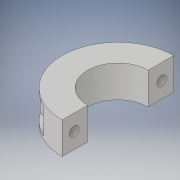
# Autodesk Inventor part: 000.402 - Зажим подшипника
Saved by Autodesk Inventor 2019 (Build 230136000, 136)
## iProperties
Created: 2020-02-28
Part Number: 000.402 - Зажим подшипника
Material: Типовые
Document SubType Name: Modeling
Designer: Петров Иван
Density: 1 g/cm^3
Appearance: По умолчанию
Author: Петров Иван
Autodesk Inventor part; units mm, degrees
ref_plane "YZ Plane" through (0, 0, 0) normal (1, 0, 0) x (0, 1, 0)
ref_plane "XZ Plane" through (0, 0, 0) normal (0, 1, 0) x (-1, 0, 0)
ref_plane "XY Plane" through (0, 0, 0) normal (0, 0, 1) x (1, 0, 0)
sketch "Эскиз1" plane through (0, 0, 0) normal (0, 1, 0) x (-1, 0, 0)
  circle A0 centre (0, 0) radius 9.5
  line L0 (0, -9.5) -> (0, -17.5)
  arc A1 (-7.7, -15.715) -> (-7.7, 15.715) centre (0, 0) ccw
  line L1 (0, 9.5) -> (0, 17.5)
  point P0 (0, -10)
  constraints: 6 point on circle, 4 end point, 2 centre point, 1 point on line
extrude "Выдавливание1" add sketch "Эскиз1" along normal blind 10 contours A0 L1 A1 L0
sketch "Эскиз2" plane through (0, 0, 17.5) normal (1, 0, 0) x (0, 0, -1)
  circle A0 centre (3.75, 5) radius 1.5 projected
  circle A1 centre (31.25, 5) radius 1.5 projected
  point P0 (17.5, 0)
extrude "Выдавливание2" cut sketch "Эскиз2" against normal through all
ref_plane "РабПлоскость1" through (-17.5, 0, 0) normal (1, 0, 0) x (0, 1, 0)
sketch "Эскиз3" plane through (-17.5, 0, 0) normal (1, 0, 0) x (0, 1, 0)
  line L0 (1, -17.25) -> (9, -17.25)
  line L1 (9, -17.25) -> (9, -10.25)
  line L2 (9, -10.25) -> (1, -10.25)
  line L3 (1, -10.25) -> (1, -17.25)
  circle A0 centre (5, -13.75) radius 1.5 projected
  line L4 (1, -17.25) -> (9, -10.25) construction
  line L5 (9, -17.25) -> (1, -10.25) construction
  line L6 (1, 10.25) -> (9, 10.25)
  line L7 (9, 10.25) -> (9, 17.25)
  line L8 (9, 17.25) -> (1, 17.25)
  line L9 (1, 17.25) -> (1, 10.25)
  circle A1 centre (5, 13.75) radius 1.5 projected
  line L10 (1, 10.25) -> (9, 17.25) construction
  line L11 (9, 10.25) -> (1, 17.25) construction
  point P0 (0, 0)
  dimension "d4" = 8
  dimension "d5" = 7
  dimension "d6" = 8
  dimension "d7" = 7
  constraints: 24 end point, 4 midpoint, 4 parallel, 2 horizontal, 2 perpendicular
  measures "d4" distance of L2.end L1.end
  measures "d5" distance of L1.end L0.end
  measures "d6" distance of L8.end L7.end
  measures "d7" distance of L7.end L6.end
extrude "Выдавливание3" cut sketch "Эскиз3" along normal blind 10 contours L3 L2 L1 L0 | A0 | L9 L8 L7 L6 | A1
equation "\"d6\" = d4"
equation "\"d7\" = d5"
